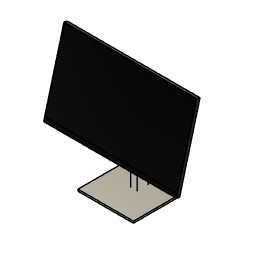
Screen-V1 (Autodesk Fusion 360 design; units mm, degrees)
Autodesk Fusion 360 part; units mm, degrees
sketch "Skizze1" plane through (0, 0, 0) normal (0, 0, 1) x (1, 0, 0)
  line L0 (-25, 15) -> (230, 15)
  line L1 (230, 15) -> (230, -190)
  line L2 (230, -190) -> (-25, -190)
  line L3 (-25, -190) -> (-25, 15)
  line L4 (87.5, -10) -> (117.5, -10)
  line L5 (117.5, -10) -> (117.5, -60)
  line L6 (117.5, -60) -> (87.5, -60)
  line L7 (87.5, -60) -> (87.5, -10)
  dimension "d1" = 255
  dimension "d2" = 205
  dimension "d3" = 30
  dimension "d4" = 50
  dimension "d5" = 25
  dimension "d6" = 112.5
  constraint horizontal L0
  constraint vertical L1
  constraint horizontal L2
  constraint vertical L3
  constraint horizontal L4
  constraint vertical L5
  constraint horizontal L6
  constraint vertical L7
  measures "d1" distance of L0.start L0.end
  measures "d2" distance of L0.start L2.end
  measures "d3" distance of L4.start L4.end
  measures "d4" distance of L4.start L6.end
  measures "d5" distance of L0 L4
  measures "d6" distance of L1 L5
extrude "Extrusion1" add sketch "Skizze1" along normal blind 8 contours L0 L1 L2 L3 | L4 L5 L6 L7 makes body 1
sketch "Skizze2" plane through (0, -190, 0) normal (0, -1, 0) x (1, 0, 0)
  line L0 (-25, 0) -> (230, 0)
  line L1 (230, 0) -> (230, 8)
  line L2 (230, 8) -> (-25, 8)
  line L3 (-25, 8) -> (-25, 0)
  line L4 (-202.5, 540) -> (407.5, 540)
  line L5 (407.5, 540) -> (407.5, 178)
  line L6 (407.5, 178) -> (-202.5, 178)
  line L7 (-202.5, 178) -> (-202.5, 540)
  dimension "d10" = 610
  dimension "d11" = 362
  dimension "d12" = 170
  dimension "d13" = 177.5
  dimension "d14" = 177.5
  constraint horizontal L4
  constraint vertical L5
  constraint horizontal L6
  constraint vertical L7
  measures "d10" distance of L4.start L4.end
  measures "d11" distance of L4.end L5.end
  measures "d12" distance of L2 L6
  measures "d13" horizontal distance of L2.end L6.end
  measures "d14" distance of L1.end L5
extrude "Extrusion2" add sketch "Skizze2" along normal blind 15 separate body contours L4 L5 L6 L7 makes body 2
move_body "Verschieben1" bodies 2 to x (1, 0, 0) y (0, 1, 0) z (0, 0, 1) at (0, 15, 0)
move_body "Verschieben2" bodies 2 to x (1, 0, 0) y (0, 0.965926, -0.258819) z (0, 0.258819, 0.965926) at (0, -52.5439, -43.1104)
move_body "Verschieben3" bodies 2 to x (1, 0, 0) y (0, 1, 0) z (0, 0, 1) at (0, 20, 0)
move_body "Verschieben4" bodies 2 to x (1, 0, 0) y (0, 1, 0) z (0, 0, 1) at (0, 30, 0)
extrude "Extrusion3" add sketch "Skizze1" along normal blind 388 separate body contours L4 L5 L6 L7 makes body 3
move_body "Verschieben5" bodies 2 to x (1, 0, 0) y (0, 1, 0) z (0, 0, 1) at (0, -30, 0)
sketch "Skizze3" plane through (0, -60, 0) normal (0, -1, 0) x (1, 0, 0)
  line L0 (87.5, 0) -> (117.5, 0)
  line L1 (117.5, 0) -> (117.5, 388)
  line L2 (117.5, 388) -> (87.5, 388)
  line L3 (87.5, 388) -> (87.5, 0)
  line L4 (87.5, 388) -> (117.5, 388)
  line L5 (117.5, 388) -> (117.5, 348)
  line L6 (117.5, 348) -> (87.5, 348)
  line L7 (87.5, 348) -> (87.5, 388)
  dimension "d19" = 40
  constraint horizontal L4
  constraint vertical L5
  constraint horizontal L6
  constraint vertical L7
  constraint coincident L1 L5.end
  constraint coincident L2.end L3.start
  measures "d19" distance of L1.end L5.end
extrude "Extrusion4" add sketch "Skizze3" along normal blind 55 separate body contours L1 L2 L3 L4 L5 L6 L7 makes body 4
ref_plane "Arbeitsebene1" through (102.5, -108.6649, 348.9503) normal (0, 0.965926, -0.258819) x (-1, 0, 0)
split "Teilen1" by plane through (102.5, -108.6649, 348.9503) normal (0, 0.965926, -0.258819) bodies 4 makes body 5 at (117.5, -89.0403, 361.3333)
delete_body "Körper entfernen1" bodies 4
sketch "Skizze4" plane through (0, -203.1122, 54.4237) normal (0, -0.965926, 0.258819) x (1, 0, 0)
  line L0 (-202.5, 127.9356) -> (407.5, 127.9356)
  line L1 (407.5, 127.9356) -> (407.5, 489.9356)
  line L2 (407.5, 489.9356) -> (-202.5, 489.9356)
  line L3 (-202.5, 489.9356) -> (-202.5, 127.9356)
  line L4 (-200.5, 487.9356) -> (405.5, 487.9356)
  line L5 (405.5, 487.9356) -> (405.5, 145.9356)
  line L6 (405.5, 145.9356) -> (-200.5, 145.9356)
  line L7 (-200.5, 145.9356) -> (-200.5, 487.9356)
  dimension "d25" = 2
  dimension "d26" = 2
  dimension "d27" = 2
  dimension "d28" = 18
  constraint horizontal L4
  constraint vertical L5
  constraint horizontal L6
  constraint vertical L7
  measures "d25" distance of L1 L5
  measures "d26" distance of L3 L7
  measures "d27" distance of L2 L4
  measures "d28" distance of L0 L6
extrude "Extrusion6" cut sketch "Skizze4" against normal blind 0.01 contours L4 L5 L6 L7 bodies 2
equation "d17 = 380 mm + 8 mm"
named bodies: "baseplate", "screen", "stand", "stand-arm"
